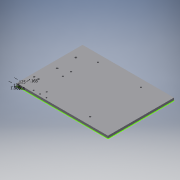
# Autodesk Inventor part: Plexiglass Hub Holding Plate
Saved by Autodesk Inventor 2019 (Build 230136000, 136)
## iProperties
Created: 2019-02-04
Part Number: Plexiglass Hub Holding Plate
Material: Generic
Document SubType Name: Modeling
Designer: mrhftc
Density: 1 g/cm^3
Appearance: Default
Author: mrhftc
Autodesk Inventor part; units mm, degrees
ref_plane "YZ Plane" through (0, 0, 0) normal (1, 0, 0) x (0, 1, 0)
ref_plane "XZ Plane" through (0, 0, 0) normal (0, 1, 0) x (-1, 0, 0)
ref_plane "XY Plane" through (0, 0, 0) normal (0, 0, 1) x (1, 0, 0)
sketch "Sketch1" plane through (0, 0, 0) normal (0, 1, 0) x (-1, 0, 0)
  line L0 (58.1245, 108.1229) -> (-170.4755, 108.1229)
  line L1 (-170.4755, 108.1229) -> (-170.4755, -56.9771)
  line L2 (-170.4755, -56.9771) -> (58.1245, -56.9771)
  line L3 (58.1245, -56.9771) -> (58.1245, 108.1229)
  circle A0 centre (-106.9755, 89.0729) radius 2.1
  circle A1 centre (-106.9755, -37.9271) radius 2.1
  constraints: 8 end point, 2 centre point, 2 parallel, 1 horizontal, 1 perpendicular
extrude "Extrusion2" add sketch "Sketch1" along normal blind 6.35
sketch "Sketch2" plane through (0, 6.35, 0) normal (0, 1, 0) x (1, 0, 0)
  circle A0 centre (-0.9745, -89.5682) radius 2.1164
  circle A1 centre (-0.9745, 38.4224) radius 2.1164
  line L0 (-58.1245, 56.9771) -> (-58.1245, -108.1229) construction
  point P0 (0, 0)
  dimension "d19" = 127.9906
  dimension "d20" = 57.15
  constraints: 2 centre point
  measures "d19" distance of A1.centre A0.centre
  measures "d20" distance from line of L0 A1.centre
extrude "Extrusion3" cut sketch "Sketch2" against normal through all
sketch "Sketch3" plane through (0, 0, 0) normal (0, -1, 0) x (1, 0, 0)
  line L0 (-58.1245, 108.1229) -> (170.4755, 108.1229) construction
  line L1 (-58.1245, -56.9771) -> (-58.1245, 108.1229) construction
  line L2 (170.4755, -56.9771) -> (-58.1245, -56.9771) construction
  circle A0 centre (-39.0745, -21.0491) radius 2.5
  circle A1 centre (-39.0745, 72.1949) radius 2.5
  circle A2 centre (-39.0745, 25.5729) radius 2.5
  point P0 (0, 0)
  dimension "d21" = 5
  dimension "d22" = 5
  dimension "d24" = 165.1
  dimension "d25" = 35.928
  dimension "d28" = 19.05
  dimension "d34" = 35.928
  constraints: 3 centre point
  measures "d21" diameter of A0
  measures "d22" diameter of A1
  measures "d24" distance between parallel lines of L0 L2
  measures "d25" distance from line of L2 A0.centre
  measures "d28" distance from line of L1 A0.centre
  measures "d34" distance from line of L0 A1.centre
extrude "Extrusion6" cut sketch "Sketch3" against normal through all
sketch "Sketch5" plane through (0, 6.35, 0) normal (0, 1, 0) x (1, 0, 0)
  line L0 (-58.1245, -108.1229) -> (170.4755, -108.1229) construction
  line L1 (170.4755, 56.9771) -> (-58.1245, 56.9771) construction
  line L2 (-58.1245, 56.9771) -> (-58.1245, -108.1229) construction
  circle A0 centre (-14.4655, -35.7769) radius 2.0955
  circle A1 centre (-14.4655, -15.3689) radius 2.0955
  line L3 (-8.4587, -93.3037) -> (-8.4587, -42.9623)
  point P0 (0, 0)
  dimension "d37" = 72.346
  dimension "d39" = 72.346
  dimension "d40" = 4.191
  dimension "d41" = 43.659
  dimension "d42" = 4.191
  dimension "d43" = 43.659
  constraints: 2 centre point, 2 end point, 1 vertical
  measures "d37" distance from line of L1 A1.centre
  measures "d39" distance from line of L0 A0.centre
  measures "d40" diameter of A1
  measures "d41" distance from line of L2 A0.centre
  measures "d42" diameter of A0
  measures "d43" distance from line of L2 A1.centre
extrude "Extrusion7" cut sketch "Sketch5" against normal through all
sketch "Sketch6" plane through (0, 0, 0) normal (0, -1, 0) x (1, 0, 0)
  line L0 (-58.1245, 108.1229) -> (170.4755, 108.1229) construction
  circle A0 centre (-20.692, 102.6189) radius 1.85
  circle A1 centre (11.308, 102.6189) radius 1.85
  circle A2 centre (-4.692, 102.6189) radius 1.85
  point P0 (0, 0)
  constraints: 3 centre point
extrude "Extrusion8" cut sketch "Sketch6" against normal through all
sketch "Sketch8" plane through (0, 0, 0) normal (0, -1, 0) x (1, 0, 0)
  line L0 (-58.1245, 108.1229) -> (170.4755, 108.1229) construction
  line L1 (-58.1245, -56.9771) -> (-58.1245, 108.1229) construction
  circle A0 centre (-54.9495, 104.5779) radius 2.1
  circle A1 centre (-54.9495, 70.0189) radius 2.1
  point P0 (0, 0)
  dimension "d53" = 4.2
  dimension "d54" = 4.2
  dimension "d55" = 3.545
  dimension "d56" = 3.175
  dimension "d57" = 3.175
  dimension "d58" = 38.104
  constraints: 2 centre point
  measures "d53" diameter of A1
  measures "d54" diameter of A0
  measures "d55" distance from line of L0 A0.centre
  measures "d56" distance from line of L1 A0.centre
  measures "d57" distance from line of L1 A1.centre
  measures "d58" distance from line of L0 A1.centre
extrude "Extrusion9" cut sketch "Sketch8" against normal through all
body "Solid2"
